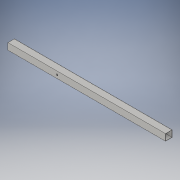
# Autodesk Inventor part: catapultArm
Saved by Autodesk Inventor 2016 SP1 (Build 200210100, 210)
## iProperties
Created: 2016-01-12
Part Number: catapultArm
Material: Generic
Document SubType Name: Modeling
Designer: steele
Density: 1 g/cm^3
Appearance: Default
Author: steele
Autodesk Inventor part; units mm, degrees
ref_plane "YZ Plane" through (0, 0, 0) normal (1, 0, 0) x (0, 1, 0)
ref_plane "XZ Plane" through (0, 0, 0) normal (0, 1, 0) x (-1, 0, 0)
ref_plane "XY Plane" through (0, 0, 0) normal (0, 0, 1) x (1, 0, 0)
sketch "Sketch1" plane through (0, 0, 0) normal (1, 0, 0) x (0, 1, 0)
  line L0 (-23.8125, 23.8125) -> (-23.8125, -23.8125)
  line L1 (-23.8125, -23.8125) -> (23.8125, -23.8125)
  line L2 (23.8125, -23.8125) -> (23.8125, 23.8125)
  line L3 (23.8125, 23.8125) -> (-23.8125, 23.8125)
  line L4 (-23.8125, 23.8125) -> (23.8125, -23.8125) construction
  line L5 (-23.8125, -23.8125) -> (23.8125, 23.8125) construction
  line L6 (-25.4, 25.4) -> (-25.4, -25.4)
  line L7 (-25.4, -25.4) -> (25.4, -25.4)
  line L8 (25.4, -25.4) -> (25.4, 25.4)
  line L9 (25.4, 25.4) -> (-25.4, 25.4)
  line L10 (-25.4, 25.4) -> (25.4, -25.4) construction
  line L11 (-25.4, -25.4) -> (25.4, 25.4) construction
  point P0 (0, 0)
  dimension "d0" = 50.8
  dimension "d1" = 1.5875
  constraints: 24 end point, 5 parallel, 4 midpoint, 4 perpendicular, 1 vertical
  measures "d0" distance of L7.end L8.end
  measures "d1" distance between parallel lines of L0 L6
extrude "Extrusion1" add sketch "Sketch1" along normal mid plane 1219.2
sketch "Sketch2" plane through (-609.6, -25.4, 25.4) normal (0, 0, 1) x (1, 0, 0)
  circle A0 centre (381, 25.4) radius 6.35
  line L0 (0, 0) -> (0, 50.8) projected
  point P0 (609.6, 25.4)
  dimension "d4" = 12.7
  dimension "d5" = 381
  constraints: 1 centre point
  measures "d4" diameter of A0
  measures "d5" distance from line of A0.centre L0
extrude "Extrusion2" cut sketch "Sketch2" against normal through all
equation "\"d0\" = catapultArmWidth"
equation "\"d1\" = catapultArmWallThickness"
equation "\"d2\" = catapultArmLength"
equation "\"d4\" = catapultArmAxelHoleDaim"
equation "\"d5\" = catapultArmHoleDistanceFromEnd"
equation "\"d6\" = catapultArmLength"
equation "\"catapultArmWallThickness\" = 1.5875"
equation "\"catapultArmWidth\" = 50.8"
equation "\"catapultArmLength\" = 1219.2"
equation "\"catapultArmAxelHoleDaim\" = 12.7"
equation "\"catapultArmHoleDistanceFromEnd\" = 381"
body "Solid1"
